Autodesk Inventor part; units mm, degrees
note: some values were not read from the file. Chosen so that the rebuilt part matches the saved one: direction of "Hole2".
(part 16 of 20)
  ellipse E344 centre (-9.843752, -15.647014) end of major axis (-9.7704, -15.822284) minor radius 0.172083 (-9.728588, -15.796415) -> (-9.668946, -15.655192) ccw
  ellipse E345 centre (-10.850532, -15.747299) end of major axis (-10.841654, -15.557507) minor radius 0.073999 (-10.924833, -15.778395) -> (-10.914737, -15.859463) ccw
  ellipse E346 centre (-10.901535, -13.717011) end of major axis (-10.892656, -13.527218) minor radius 0.073999 (-10.972145, -13.675357) -> (-10.975835, -13.748106) ccw
  line L433 (-10.732194, -13.203469) -> (-10.766856, -11.823661)
  line L434 (-10.84586, -11.667497) -> (-11.030789, -11.744892)
  line L435 (-11.144186, -17.767984) -> (-10.697309, -17.58096)
  line L436 (-10.627713, -17.362604) -> (-10.662375, -15.982796)
  line L437 (-10.594189, -13.209925) -> (-10.628851, -11.830117)
  line L438 (-10.489708, -17.369061) -> (-10.52437, -15.989253)
  line L439 (-11.411804, -17.944199) -> (-10.559304, -17.587416)
  ellipse E347 centre (-10.841156, -11.854757) end of major axis (-10.832277, -11.664964) minor radius 0.073999 (-10.766856, -11.823661) -> (-10.84586, -11.667497) ccw
  ellipse E348 centre (-10.702013, -17.3937) end of major axis (-10.710892, -17.583493) minor radius 0.073999 (-10.697309, -17.58096) -> (-10.627713, -17.362604) ccw
  ellipse E349 centre (-10.703151, -11.861213) end of major axis (-10.694272, -11.671421) minor radius 0.073999 (-10.628851, -11.830117) -> (-10.694272, -11.671421) ccw
  ellipse E350 centre (-10.564008, -17.400156) end of major axis (-10.572887, -17.589949) minor radius 0.073999 (-10.559304, -17.587416) -> (-10.489708, -17.369061) ccw
  line L440 (-10.832277, -11.664964) -> (-10.694272, -11.671421)
  line L441 (-10.643313, -18.02564) -> (-11.279559, -17.995875)
  line L442 (-11.338217, -18.020424) -> (-10.641932, -18.052998)
  ellipse E351 centre (-11.181795, -17.954959) end of major axis (-11.431717, -17.961237) minor radius 0.041852 (-11.411804, -17.944199) -> (-11.279559, -17.995875) ccw
  ellipse E352 centre (-11.181795, -17.954959) end of major axis (-11.581669, -17.965004) minor radius 0.066962 (-11.579808, -17.958216) -> (-11.338217, -18.020424) ccw
  line L443 (-11.581818, -17.959094) -> (-11.581669, -17.965004)
  line L444 (9.445486, -13.382673) -> (9.726407, -13.372264)
  line L445 (9.577459, -15.622189) -> (9.444613, -14.35264)
  ellipse E353 centre (9.612924, -11.790422) end of major axis (9.588034, -11.602059) minor radius 0.101721 (9.69231, -11.695037) -> (9.593168, -11.601626) ccw
  line L446 (9.593168, -11.601626) -> (9.489906, -11.605452)
  line L447 (9.680903, -17.583459) -> (9.975636, -17.572538)
  line L448 (9.986075, -17.572152) -> (10.054617, -17.569612)
  line L449 (9.494074, -17.602324) -> (9.600374, -17.598385)
  ellipse E354 centre (9.679434, -15.618411) end of major axis (9.704324, -15.806773) minor radius 0.101721 (9.577459, -15.622189) -> (9.667019, -15.799296) ccw
  ellipse E355 centre (9.465242, -13.571468) end of major axis (9.440352, -13.383106) minor radius 0.101721 (9.445486, -13.382673) -> (9.445133, -13.382687) ccw
  line L450 (-9.369641, -11.620465) -> (-9.45962, -11.620315)
  line L451 (-9.704796, -17.582819) -> (-9.665179, -17.582885)
  line L452 (-9.476199, -17.583199) -> (-9.245372, -17.583582)
  line L453 (-9.152463, -17.394911) -> (-9.079808, -16.701606)
  line L454 (-9.581549, -17.599678) -> (-9.512402, -17.599793)
  ellipse E356 centre (-9.225588, -17.39479) end of major axis (-9.248733, -17.583375) minor radius 0.072673 (-9.245372, -17.583582) -> (-9.152463, -17.394911) ccw
  line L455 (-9.214159, -15.814637) -> (-9.257838, -15.814565)
  ellipse E357 centre (-9.092788, -11.665336) end of major axis (-9.49061, -11.623647) minor radius 0.017093 (-9.45962, -11.620315) -> (-9.49061, -11.623647) ccw
  line L456 (-9.49061, -11.623647) -> (-9.491123, -11.628548)
  line L457 (11.417851, -17.944787) -> (11.028639, -17.977434)
  line L458 (10.650943, -18.039039) -> (11.499343, -17.967874)
  ellipse E358 centre (11.422583, -17.757528) end of major axis (11.370793, -17.940333) minor radius 0.156811 (11.417851, -17.944787) -> (11.502296, -17.909857) ccw
  ellipse E359 centre (11.504076, -17.780615) end of major axis (11.452286, -17.963421) minor radius 0.156811 (11.499343, -17.967874) -> (11.586117, -17.931064) ccw
  line L459 (10.678705, -11.674527) -> (10.647369, -11.665649)
  line L460 (10.497918, -17.579089) -> (10.937664, -17.703672)
  line L461 (10.490349, -17.623165) -> (11.556403, -17.925185)
  line L462 (10.603032, -13.41997) -> (10.918137, -13.509241)
  line L463 (11.016629, -13.725744) -> (10.965317, -15.756025)
  ellipse E360 centre (10.26736, -13.448126) end of major axis (10.667233, -13.458232) minor radius 0.066962 (10.603032, -13.41997) -> (10.37813, -13.386485) ccw
  line L464 (9.644854, -13.420548) -> (9.985302, -13.391991)
  ellipse E361 centre (10.26736, -13.448126) end of major axis (10.01744, -13.44181) minor radius 0.041852 (10.251549, -13.405957) -> (10.137481, -13.409169) ccw
  line L465 (10.633643, -13.474862) -> (10.568229, -13.45633)
  ellipse E362 centre (10.206584, -15.852925) end of major axis (9.806712, -15.842819) minor radius 0.066962 (10.532407, -15.822097) -> (10.256875, -15.787709) ccw
  line L466 (9.547773, -13.645477) -> (9.541369, -13.898884)
  ellipse E363 centre (10.913405, -13.6965) end of major axis (10.897523, -13.507165) minor radius 0.102463 (11.016629, -13.725744) -> (10.918137, -13.509241) ccw
  ellipse E364 centre (10.862093, -15.726781) end of major axis (10.846211, -15.537446) minor radius 0.102463 (10.937384, -15.870856) -> (10.965317, -15.756025) ccw
  ellipse E365 centre (9.707217, -13.632102) end of major axis (9.759007, -13.449297) minor radius 0.156811 (9.558959, -13.580771) -> (9.547773, -13.645477) ccw
  ellipse E366 centre (9.625724, -13.609015) end of major axis (9.573934, -13.79182) minor radius 0.156811 (9.59069, -13.430952) -> (9.493397, -13.520415) ccw
  line L467 (9.339233, -17.62641) -> (9.636108, -17.601507)
  line L468 (9.968091, -17.57366) -> (10.026426, -17.568767)
  ellipse E367 centre (10.162247, -17.607246) end of major axis (10.412167, -17.613562) minor radius 0.041852 (10.171389, -17.565634) -> (10.026426, -17.568767) ccw
  ellipse E368 centre (10.311697, -11.693806) end of major axis (9.911825, -11.6837) minor radius 0.066962 (10.647369, -11.665649) -> (10.343834, -11.627829) ccw
  ellipse E369 centre (10.162247, -17.607246) end of major axis (9.762375, -17.59714) minor radius 0.066962 (10.497918, -17.579089) -> (10.333285, -17.550901) ccw
  ellipse E370 centre (11.561135, -17.737926) end of major axis (11.577017, -17.927261) minor radius 0.102463 (11.556403, -17.925185) -> (11.575565, -17.927364) ccw
  line L469 (9.071223, -17.982215) -> (9.026913, -17.969662)
  ellipse E371 centre (-10.756466, -13.251165) end of major axis (-10.832503, -13.077043) minor radius 0.168992 (-10.928737, -13.245323) -> (-10.838461, -13.407289) ccw
  ellipse E372 centre (-10.819297, -13.278602) end of major axis (-10.74326, -13.452724) minor radius 0.168992 (-10.947502, -13.391229) -> (-10.896969, -13.437563) ccw
  ellipse E373 centre (-11.00923, -13.280047) end of major axis (-11.015669, -13.469938) minor radius 0.079929 (-10.999805, -13.46675) -> (-10.929643, -13.245292) ccw
  ellipse E374 centre (-11.145233, -13.275435) end of major axis (-11.151672, -13.465326) minor radius 0.079929 (-11.135808, -13.462138) -> (-11.065647, -13.240681) ccw
  ellipse E375 centre (-11.005348, -16.0465) end of major axis (-10.998909, -15.856609) minor radius 0.079929 (-10.925762, -16.011746) -> (-11.014773, -15.859797) ccw
  ellipse E376 centre (-10.616581, -16.02223) end of major axis (-10.692618, -15.848108) minor radius 0.168992 (-10.754817, -15.898029) -> (-10.788852, -16.016388) ccw
  ellipse E377 centre (-10.869345, -16.051112) end of major axis (-10.862906, -15.861221) minor radius 0.079929 (-10.789758, -16.016357) -> (-10.862906, -15.861221) ccw
  line L470 (-10.862906, -15.861221) -> (-10.998909, -15.856609)
  line L471 (-10.679739, -13.469718) -> (-10.756571, -13.467113)
  line L472 (-10.691215, -13.439761) -> (-10.615929, -13.442313)
  line L473 (-10.019153, -15.69929) -> (-10.037208, -15.341622)
  line L474 (-10.11165, -13.866954) -> (-10.121338, -13.675036)
  line L475 (-11.395511, -13.575548) -> (-11.135808, -13.462138)
  line L476 (-10.999805, -13.46675) -> (-11.259507, -13.580159)
  line L477 (-12.048956, -13.860901) -> (-11.806008, -13.754808)
  line L478 (-11.716997, -13.906757) -> (-11.614811, -15.93101)
  line L479 (-11.684973, -16.152467) -> (-11.92792, -16.25856)
  line L480 (-11.014773, -15.859797) -> (-11.274475, -15.973207)
  line L481 (-11.363486, -15.821258) -> (-11.465672, -13.797005)
  line L482 (-10.540849, -15.838414) -> (-10.571702, -15.837368)
  line L483 (-11.329669, -13.801617) -> (-11.227483, -15.82587)
  ellipse E378 centre (-11.68628, -13.873199) end of major axis (-12.085772, -13.893366) minor radius 0.071491 (-12.048956, -13.860901) -> (-11.85383, -13.946367) ccw
  line L484 (-11.714759, -13.951082) -> (-11.85383, -13.946367)
  line L485 (-11.790999, -13.918929) -> (-11.733349, -13.920884)
  ellipse E379 centre (-11.68628, -13.873199) end of major axis (-11.935962, -13.885803) minor radius 0.044682 (-11.912952, -13.865513) -> (-11.790999, -13.918929) ccw
  line L486 (-11.743379, -13.791462) -> (-11.912952, -13.865513)
  ellipse E380 centre (-11.565245, -16.270858) end of major axis (-11.964736, -16.291025) minor radius 0.071491 (-11.92792, -16.25856) -> (-11.964736, -16.291025) ccw
  line L487 (-10.058507, -13.647599) -> (-10.044208, -13.930851)
  line L488 (-9.974022, -15.321217) -> (-9.956321, -15.671852)
  ellipse E381 centre (-10.888744, -11.902896) end of major axis (-10.964781, -11.728775) minor radius 0.168992 (-10.964781, -11.728775) -> (-11.018932, -11.768677) ccw
  ellipse E382 centre (-10.609966, -17.425373) end of major axis (-10.533929, -17.599495) minor radius 0.168992 (-10.615379, -17.610884) -> (-10.600541, -17.612076) ccw
  ellipse E383 centre (-10.547135, -17.397936) end of major axis (-10.623172, -17.223814) minor radius 0.168992 (-10.552098, -17.583502) -> (-10.53771, -17.584639) ccw
  ellipse E384 centre (-10.547135, -17.397936) end of major axis (-10.623172, -17.223814) minor radius 0.168992 (-10.719405, -17.392094) -> (-10.702191, -17.465134) ccw
  ellipse E385 centre (-10.825913, -11.875459) end of major axis (-10.90195, -11.701337) minor radius 0.168992 (-10.895835, -11.698825) -> (-10.998183, -11.869617) ccw
  line L489 (-10.964781, -11.728775) -> (-10.90195, -11.701337)
  line L490 (-10.600541, -17.612076) -> (-10.583907, -17.61264)
  line L491 (-10.431975, -17.617792) -> (-9.338389, -17.654875)
  line L492 (-10.719405, -17.392094) -> (-10.788852, -16.016388)
  line L493 (-10.266545, -17.593834) -> (-10.349114, -17.591034)
  line L494 (-10.517241, -17.585333) -> (-10.53771, -17.584639)
  line L495 (-10.661005, -11.694667) -> (-10.643146, -11.695273)
  line L496 (-10.928737, -13.245323) -> (-10.998183, -11.869617)
  ellipse E386 centre (-10.191423, -15.693448) end of major axis (-10.115386, -15.86757) minor radius 0.168992 (-10.03213, -15.779735) -> (-10.019153, -15.69929) ccw
  ellipse E387 centre (-10.293609, -13.669195) end of major axis (-10.217572, -13.843316) minor radius 0.168992 (-10.121338, -13.675036) -> (-10.128707, -13.629799) ccw
  ellipse E388 centre (-11.796583, -13.941511) end of major axis (-11.790144, -13.75162) minor radius 0.079929 (-11.716997, -13.906757) -> (-11.806008, -13.754808) ccw
  ellipse E389 centre (-11.694398, -15.965764) end of major axis (-11.700837, -16.155655) minor radius 0.079929 (-11.684973, -16.152467) -> (-11.614811, -15.93101) ccw
  ellipse E390 centre (-11.2839, -15.786504) end of major axis (-11.290339, -15.976395) minor radius 0.079929 (-11.363486, -15.821258) -> (-11.274475, -15.973207) ccw
  ellipse E391 centre (-11.386086, -13.762251) end of major axis (-11.379647, -13.57236) minor radius 0.079929 (-11.395511, -13.575548) -> (-11.465672, -13.797005) ccw
  ellipse E392 centre (-10.230778, -13.641757) end of major axis (-10.306815, -13.467635) minor radius 0.168992 (-10.058507, -13.647599) -> (-10.064377, -13.608062) ccw
  ellipse E393 centre (-10.128592, -15.66601) end of major axis (-10.204629, -15.491889) minor radius 0.168992 (-9.990742, -15.79073) -> (-9.956321, -15.671852) ccw
  ellipse E394 centre (-11.147897, -15.791116) end of major axis (-11.141458, -15.601225) minor radius 0.079929 (-11.227483, -15.82587) -> (-11.201101, -15.941165) ccw
  ellipse E395 centre (-11.250082, -13.766862) end of major axis (-11.243643, -13.576972) minor radius 0.079929 (-11.259507, -13.580159) -> (-11.329669, -13.801617) ccw
  line L497 (-11.065647, -13.240681) -> (-11.135093, -11.864974)
  line L498 (-11.224104, -11.713026) -> (-12.137252, -12.111789)
  line L499 (-11.839624, -18.007672) -> (-10.926477, -17.608909)
  line L500 (-10.856315, -17.387452) -> (-10.925762, -16.011746)
  line L501 (-10.929643, -13.245292) -> (-10.99909, -11.869586)
  line L502 (-10.720312, -17.392063) -> (-10.789758, -16.016357)
  line L503 (-11.703621, -18.012284) -> (-10.790473, -17.613521)
  ellipse E396 centre (-11.214679, -11.899729) end of major axis (-11.20824, -11.709838) minor radius 0.079929 (-11.135093, -11.864974) -> (-11.224104, -11.713026) ccw
  ellipse E397 centre (-10.935901, -17.422206) end of major axis (-10.94234, -17.612097) minor radius 0.079929 (-10.926477, -17.608909) -> (-10.856315, -17.387452) ccw
  ellipse E398 centre (-11.078676, -11.904341) end of major axis (-11.072237, -11.71445) minor radius 0.079929 (-10.99909, -11.869586) -> (-11.072237, -11.71445) ccw
  ellipse E399 centre (-10.799898, -17.426818) end of major axis (-10.806337, -17.616709) minor radius 0.079929 (-10.790473, -17.613521) -> (-10.720312, -17.392063) ccw
  line L504 (-11.20824, -11.709838) -> (-11.072237, -11.71445)
  line L505 (-10.639678, -18.097642) -> (-11.581668, -18.0657)
  line L506 (-11.644499, -18.093138) -> (-10.638183, -18.127261)
  ellipse E400 centre (-11.476949, -18.01997) end of major axis (-11.726631, -18.032574) minor radius 0.044682 (-11.703621, -18.012284) -> (-11.581668, -18.0657) ccw
  ellipse E401 centre (-11.774577, -12.124087) end of major axis (-12.174068, -12.144254) minor radius 0.071491 (-12.137252, -12.111789) -> (-12.174068, -12.144254) ccw
  ellipse E402 centre (-11.476949, -18.01997) end of major axis (-11.87644, -18.040137) minor radius 0.071491 (-11.839624, -18.007672) -> (-11.644499, -18.093138) ccw
  line L507 (-12.174068, -12.144254) -> (-12.085772, -13.893366)
  line L508 (-11.964736, -16.291025) -> (-11.87644, -18.040137)
  ellipse E403 centre (9.621764, -13.167497) end of major axis (9.645394, -13.356022) minor radius 0.095931 (9.643038, -13.356259) -> (9.717505, -13.160222) ccw
  line L509 (9.645394, -13.356022) -> (9.618841, -13.35935)
  line L510 (9.443815, -13.371397) -> (9.643038, -13.356259)
  line L511 (9.799774, -15.789209) -> (9.60382, -15.804099)
  line L512 (9.486806, -15.622612) -> (9.386714, -14.734494)
  line L513 (9.717505, -13.160222) -> (9.560751, -11.769345)
  line L514 (9.443737, -11.587858) -> (9.2374, -11.603537)
  line L515 (9.01704, -17.632231) -> (9.957912, -17.560738)
  line L516 (8.945553, -17.644004) -> (9.57653, -17.596058)
  ellipse E404 centre (9.46501, -11.77662) end of major axis (9.441381, -11.588095) minor radius 0.095931 (9.560751, -11.769345) -> (9.443737, -11.587858) ccw
  ellipse E405 centre (9.582546, -15.615337) end of major axis (9.606176, -15.803862) minor radius 0.095931 (9.486806, -15.622612) -> (9.60382, -15.804099) ccw
  ellipse E406 centre (8.67445, -17.675171) end of major axis (8.276966, -17.719968) minor radius 0.00852 (9.01704, -17.632231) -> (8.94642, -17.638281) ccw
  line L517 (-9.228619, -11.605746) -> (-9.331213, -11.599017)
  line L518 (-9.855856, -17.569528) -> (-9.103656, -17.618867)
  line L519 (-9.00389, -17.435255) -> (-8.988858, -17.302054)
  line L520 (-9.540587, -17.597944) -> (-8.968083, -17.635496)
  line L521 (-9.530783, -13.367387) -> (-9.435311, -13.373649)
  line L522 (-9.370298, -14.783825) -> (-9.465065, -15.623544)
  line L523 (-9.564831, -15.807156) -> (-9.804351, -15.791446)
  ellipse E407 centre (-9.169255, -13.411732) end of major axis (-9.566732, -13.366875) minor radius 0.00852 (-9.530783, -13.367387) -> (-9.557888, -13.366094) ccw
  ellipse E408 centre (-9.442823, -15.83579) end of major axis (-9.8403, -15.790933) minor radius 0.00852 (-9.804351, -15.791446) -> (-9.8403, -15.790933) ccw
  ellipse E409 centre (-9.543528, -15.618398) end of major axis (-9.56666, -15.806984) minor radius 0.078528 (-9.564831, -15.807156) -> (-9.465065, -15.623544) ccw
  ellipse E410 centre (-9.082354, -17.430108) end of major axis (-9.105486, -17.618695) minor radius 0.078528 (-9.103656, -17.618867) -> (-9.00389, -17.435255) ccw
  ellipse E411 centre (-8.946781, -17.446738) end of major axis (-8.969913, -17.635324) minor radius 0.078528 (-8.968083, -17.635496) -> (-8.939824, -17.625771) ccw
  ellipse E412 centre (-8.969685, -11.643361) end of major axis (-9.367162, -11.598504) minor radius 0.00852 (-9.331213, -11.599017) -> (-9.367162, -11.598504) ccw
  line L524 (-9.367162, -11.598504) -> (-9.370271, -11.626052)
  line L525 (-9.8403, -15.790933) -> (-9.841486, -15.80144)
  ellipse E413 centre (11.975018, -13.723987) end of major axis (11.912145, -13.903283) minor radius 0.159857 (11.965565, -13.910689) -> (12.063067, -13.869699) ccw
  ellipse E414 centre (11.898512, -13.697159) end of major axis (11.835639, -13.876455) minor radius 0.159857 (11.889059, -13.88386) -> (11.979456, -13.848629) ccw
  ellipse E415 centre (12.042124, -13.680589) end of major axis (12.053014, -13.870276) minor radius 0.096916 (12.032671, -13.86729) -> (12.053014, -13.870276) ccw
  ellipse E416 centre (12.170931, -13.673194) end of major axis (12.181821, -13.862882) minor radius 0.096916 (12.161477, -13.859896) -> (12.267838, -13.707176) ccw
  ellipse E417 centre (12.030624, -16.444238) end of major axis (12.019734, -16.25455) minor radius 0.096916 (12.127532, -16.47822) -> (12.040078, -16.257536) ccw
  line L526 (12.181821, -13.862882) -> (12.053014, -13.870276)
  line L527 (11.796803, -13.889157) -> (11.889059, -13.88386)
  line L528 (11.965565, -13.910689) -> (11.749956, -13.923067)
  line L529 (11.845253, -13.749005) -> (12.161477, -13.859896)
  line L530 (12.032671, -13.86729) -> (11.775728, -13.777188)
  line L531 (11.049591, -13.469992) -> (11.345414, -13.573728)
  line L532 (11.432868, -13.794412) -> (11.330375, -15.818649)
  line L533 (11.224014, -15.971368) -> (10.928191, -15.867632)
  line L534 (12.040078, -16.257536) -> (11.723853, -16.146646)
  line L535 (11.636399, -15.925962) -> (11.738892, -13.901725)
  ellipse E418 centre (10.706106, -13.489711) end of major axis (11.105595, -13.509938) minor radius 0.071491 (11.049591, -13.469992) -> (10.616703, -13.415564) ccw
  ellipse E419 centre (10.706106, -13.489711) end of major axis (10.456426, -13.477069) minor radius 0.044682 (10.920784, -13.477386) -> (10.707082, -13.445022) ccw
  line L536 (11.216607, -13.581122) -> (10.920784, -13.477386)
  ellipse E420 centre (10.584706, -15.887352) end of major axis (10.185218, -15.867124) minor radius 0.071491 (10.928191, -15.867632) -> (10.492843, -15.813187) ccw
  line L537 (11.201568, -15.826044) -> (11.304061, -13.801806)
  line L538 (9.800222, -15.612006) -> (9.815689, -15.306536)
  line L539 (9.877415, -14.087452) -> (9.899198, -13.657237)
  line L540 (11.679097, -18.0306) -> (10.648374, -18.089773)
  line L541 (10.646789, -18.121084) -> (11.755603, -18.057428)
  ellipse E421 centre (11.68855, -17.843898) end of major axis (11.625676, -18.023194) minor radius 0.159857 (11.679097, -18.0306) -> (11.769494, -17.995369) ccw
  ellipse E422 centre (11.765056, -17.870726) end of major axis (11.702182, -18.050022) minor radius 0.159857 (11.755603, -18.057428) -> (11.853105, -18.016438) ccw
  line L542 (12.267838, -13.707176) -> (12.337494, -12.331481)
  line L543 (12.25004, -12.110797) -> (11.138153, -11.720893)
  line L544 (10.839628, -17.616731) -> (11.951515, -18.006635)
  line L545 (12.057876, -17.853916) -> (12.127532, -16.47822)
  line L546 (10.710822, -17.624126) -> (11.822709, -18.014029)
  ellipse E423 centre (12.240586, -12.297499) end of major axis (12.229697, -12.107811) minor radius 0.096916 (12.337494, -12.331481) -> (12.25004, -12.110797) ccw
  ellipse E424 centre (11.960969, -17.819933) end of major axis (11.971858, -18.009621) minor radius 0.096916 (11.951515, -18.006635) -> (12.057876, -17.853916) ccw
  ellipse E425 centre (11.832162, -17.827328) end of major axis (11.843052, -18.017016) minor radius 0.096916 (11.822709, -18.014029) -> (11.843052, -18.017016) ccw
  line L547 (11.971858, -18.009621) -> (11.843052, -18.017016)
  ellipse E426 centre (11.33596, -13.760429) end of major axis (11.325071, -13.570741) minor radius 0.096916 (11.432868, -13.794412) -> (11.345414, -13.573728) ccw
  ellipse E427 centre (11.233467, -15.784667) end of major axis (11.244357, -15.974354) minor radius 0.096916 (11.224014, -15.971368) -> (11.330375, -15.818649) ccw
  ellipse E428 centre (11.733306, -15.959945) end of major axis (11.744196, -16.149632) minor radius 0.096916 (11.636399, -15.925962) -> (11.723853, -16.146646) ccw
  ellipse E429 centre (11.8358, -13.935707) end of major axis (11.82491, -13.746019) minor radius 0.096916 (11.845253, -13.749005) -> (11.738892, -13.901725) ccw
  ellipse E430 centre (11.207154, -13.767824) end of major axis (11.196264, -13.578136) minor radius 0.096916 (11.304061, -13.801806) -> (11.216607, -13.581122) ccw
  ellipse E431 centre (10.139788, -13.656348) end of major axis (10.202661, -13.477052) minor radius 0.159857 (9.980403, -13.634911) -> (9.978619, -13.645423) ccw
  ellipse E432 centre (10.063282, -13.62952) end of major axis (10.000409, -13.808815) minor radius 0.159857 (9.90416, -13.606757) -> (9.901654, -13.621935) ccw
  ellipse E433 centre (9.960788, -15.653757) end of major axis (9.897915, -15.833053) minor radius 0.159857 (9.802392, -15.719049) -> (9.83254, -15.784764) ccw
  ellipse E434 centre (10.037294, -15.680585) end of major axis (10.100168, -15.50129) minor radius 0.159857 (9.876569, -15.734065) -> (9.890555, -15.780496) ccw
  ellipse E435 centre (11.10466, -15.792061) end of major axis (11.11555, -15.981749) minor radius 0.096916 (11.164732, -15.95058) -> (11.201568, -15.826044) ccw
  line L548 (9.677127, -17.631435) -> (10.306232, -17.595319)
  line L549 (10.204137, -17.56996) -> (10.003578, -17.581474)
  line L550 (9.653068, -17.601596) -> (9.595968, -17.604874)
  ellipse E436 centre (10.496144, -17.63645) end of major axis (10.745824, -17.649092) minor radius 0.044682 (10.710822, -17.624126) -> (10.579336, -17.598346) ccw
  ellipse E437 centre (10.794669, -11.740612) end of major axis (10.39518, -11.720385) minor radius 0.071491 (11.138153, -11.720893) -> (10.651336, -11.666773) ccw
  ellipse E438 centre (10.496144, -17.63645) end of major axis (10.096656, -17.616223) minor radius 0.071491 (10.839628, -17.616731) -> (10.47045, -17.563759) ccw
  ellipse E439 centre (-10.031545, -13.19179) end of major axis (-9.973156, -13.372596) minor radius 0.167961 (-10.201705, -13.17958) -> (-10.030323, -13.379423) ccw
  ellipse E440 centre (-10.098273, -13.213339) end of major axis (-10.039884, -13.394145) minor radius 0.167961 (-10.228099, -13.324234) -> (-10.097051, -13.400972) ccw
  ellipse E441 centre (-10.080134, -15.998197) end of major axis (-10.138523, -15.817391) minor radius 0.167961 (-10.138523, -15.817391) -> (-10.201976, -15.857572) ccw
  ellipse E442 centre (-10.287123, -13.206811) end of major axis (-10.300722, -13.396324) minor radius 0.083645 (-10.285901, -13.394443) -> (-10.2026, -13.179515) ccw
  ellipse E443 centre (-10.42146, -13.197171) end of major axis (-10.435059, -13.386684) minor radius 0.083645 (-10.420238, -13.384803) -> (-10.336937, -13.169875) ccw
  ellipse E444 centre (-10.403321, -15.982028) end of major axis (-10.389722, -15.792516) minor radius 0.083645 (-10.318798, -15.954733) -> (-10.404543, -15.794396) ccw
  ellipse E445 centre (-10.013406, -15.976648) end of major axis (-10.071795, -15.795842) minor radius 0.167961 (-10.014628, -15.789016) -> (-10.183566, -15.964437) ccw
  ellipse E446 centre (-10.268984, -15.991668) end of major axis (-10.255385, -15.802156) minor radius 0.083645 (-10.184461, -15.964373) -> (-10.255385, -15.802156) ccw
  line L551 (-10.071795, -15.795842) -> (-10.138523, -15.817391)
  line L552 (-10.255385, -15.802156) -> (-10.389722, -15.792516)
  line L553 (-9.596422, -13.436897) -> (-10.097051, -13.400972)
  line L554 (-10.030323, -13.379423) -> (-9.529694, -13.415348)
  line L555 (-10.696048, -13.473872) -> (-10.682857, -13.469612)
  line L556 (-10.681518, -13.46918) -> (-10.420238, -13.384803)
  line L557 (-10.285901, -13.394443) -> (-10.456104, -13.449408)
  line L558 (-10.404543, -15.794396) -> (-10.558715, -15.844184)
  line L559 (-10.766099, -15.723128) -> (-10.774361, -14.454574)
  line L560 (-10.777236, -14.013288) -> (-10.779349, -13.6888)
  line L561 (-9.75757, -15.807462) -> (-10.014628, -15.789016)
  line L562 (-10.645012, -13.69844) -> (-10.643342, -13.954818)
  line L563 (-10.634006, -15.388151) -> (-10.631762, -15.732769)
  ellipse E447 centre (-10.107278, -11.830786) end of major axis (-10.165667, -11.64998) minor radius 0.167961 (-10.165667, -11.64998) -> (-10.22912, -11.690161) ccw
  ellipse E448 centre (-10.071129, -17.38075) end of major axis (-10.012741, -17.561556) minor radius 0.167961 (-10.200955, -17.491645) -> (-10.069907, -17.568383) ccw
  ellipse E449 centre (-10.004401, -17.359201) end of major axis (-9.946012, -17.540007) minor radius 0.167961 (-10.174561, -17.346991) -> (-10.003179, -17.546834) ccw
  ellipse E450 centre (-10.04055, -11.809237) end of major axis (-10.098938, -11.628431) minor radius 0.167961 (-10.041772, -11.621605) -> (-10.21071, -11.797026) ccw
  line L564 (-10.165667, -11.64998) -> (-10.098938, -11.628431)
  line L565 (-10.069907, -17.568383) -> (-9.882923, -17.581801)
  line L566 (-9.62212, -17.600516) -> (-9.24945, -17.627259)
  line L567 (-10.174561, -17.346991) -> (-10.183566, -15.964437)
  line L568 (-9.826429, -17.559517) -> (-10.003179, -17.546834)
  line L569 (-10.041772, -11.621605) -> (-9.593855, -11.653747)
  line L570 (-10.201705, -13.17958) -> (-10.21071, -11.797026)
  ellipse E451 centre (-9.5952, -13.624529) end of major axis (-9.653589, -13.443723) minor radius 0.167961 (-9.453768, -13.531516) -> (-9.596422, -13.436897) ccw
  ellipse E452 centre (-10.681576, -15.695833) end of major axis (-10.695175, -15.885346) minor radius 0.083645 (-10.766099, -15.723128) -> (-10.754244, -15.813011) ccw
  ellipse E453 centre (-10.694826, -13.661504) end of major axis (-10.681227, -13.471992) minor radius 0.083645 (-10.696048, -13.473872) -> (-10.710578, -13.48137) ccw
  ellipse E454 centre (-10.694826, -13.661504) end of major axis (-10.708426, -13.851017) minor radius 0.083645 (-10.772841, -13.611804) -> (-10.779349, -13.6888) ccw
  ellipse E455 centre (-9.528472, -13.60298) end of major axis (-9.58686, -13.422174) minor radius 0.167961 (-9.474177, -13.429569) -> (-9.529694, -13.415348) ccw
  ellipse E456 centre (-10.547239, -15.705473) end of major axis (-10.53364, -15.51596) minor radius 0.083645 (-10.631762, -15.732769) -> (-10.626023, -15.796522) ccw
  ellipse E457 centre (-10.560489, -13.671145) end of major axis (-10.54689, -13.481632) minor radius 0.083645 (-10.638486, -13.62134) -> (-10.645012, -13.69844) ccw
  line L571 (-10.336937, -13.169875) -> (-10.345942, -11.787322)
  line L572 (-10.431687, -11.626985) -> (-10.657434, -11.699887)
  line L573 (-10.752585, -17.668307) -> (-10.393094, -17.552214)
  line L574 (-10.309793, -17.337287) -> (-10.318798, -15.954733)
  line L575 (-10.2026, -13.179515) -> (-10.211605, -11.796962)
  line L576 (-10.175456, -17.346927) -> (-10.184461, -15.964373)
  line L577 (-11.228543, -17.875033) -> (-10.258757, -17.561854)
  ellipse E458 centre (-10.430465, -11.814617) end of major axis (-10.416865, -11.625105) minor radius 0.083645 (-10.345942, -11.787322) -> (-10.431687, -11.626985) ccw
  ellipse E459 centre (-10.394316, -17.364582) end of major axis (-10.407915, -17.554095) minor radius 0.083645 (-10.393094, -17.552214) -> (-10.309793, -17.337287) ccw
  ellipse E460 centre (-10.296128, -11.824257) end of major axis (-10.282529, -11.634745) minor radius 0.083645 (-10.211605, -11.796962) -> (-10.282529, -11.634745) ccw
  ellipse E461 centre (-10.259979, -17.374222) end of major axis (-10.273578, -17.563735) minor radius 0.083645 (-10.258757, -17.561854) -> (-10.175456, -17.346927) ccw
  line L578 (-10.416865, -11.625105) -> (-10.282529, -11.634745)
  line L579 (-10.993106, -17.935823) -> (-11.115863, -17.927014)
  line L580 (-11.182591, -17.948563) -> (-10.961458, -17.964432)
  ellipse E462 centre (-11.004649, -17.891099) end of major axis (-11.254643, -17.892728) minor radius 0.039312 (-11.228543, -17.875033) -> (-11.115863, -17.927014) ccw
  ellipse E463 centre (-11.004649, -17.891099) end of major axis (-10.604657, -17.888494) minor radius 0.062899 (-11.359601, -17.922351) -> (-11.182591, -17.948563) ccw
  line L581 (9.569097, -13.392619) -> (9.66923, -13.393144)
  line L582 (9.560898, -13.410165) -> (9.53155, -13.410011)
  line L583 (9.69419, -15.627786) -> (9.494388, -13.58092)
  ellipse E464 centre (9.718804, -11.81435) end of major axis (9.694287, -11.625939) minor radius 0.092496 (9.718615, -11.629173) -> (9.700376, -11.625561) ccw
  ellipse E465 centre (10.133966, -17.415425) end of major axis (10.158483, -17.603837) minor radius 0.092496 (10.152394, -17.604214) -> (10.158483, -17.603837) ccw
  line L584 (10.15897, -17.603773) -> (10.158483, -17.603837)
  line L585 (9.700376, -11.625561) -> (9.647072, -11.625282)
  line L586 (9.712882, -17.584322) -> (10.015932, -17.58591)
  line L587 (9.530976, -17.600956) -> (9.91367, -17.602962)
  line L588 (10.151389, -17.604208) -> (10.152394, -17.604214)
  ellipse E466 centre (9.787328, -15.628274) end of major axis (9.811845, -15.816685) minor radius 0.092496 (9.69419, -15.627786) -> (9.756335, -15.791118) ccw
  ellipse E467 centre (9.587526, -13.581408) end of major axis (9.563009, -13.392996) minor radius 0.092496 (9.569097, -13.392619) -> (9.494388, -13.58092) ccw
  line L589 (-9.364516, -11.625933) -> (-9.601494, -11.630827)
  line L590 (-9.934587, -17.587325) -> (-9.692602, -17.582328)
  line L591 (-9.826588, -17.604738) -> (-9.571711, -17.599475)
  line L592 (-9.659339, -13.397075) -> (-9.51984, -13.394194)
  line L593 (-9.493169, -13.972646) -> (-9.655017, -15.628093)
  line L594 (-9.484689, -13.413112) -> (-9.525115, -13.413947)
  ellipse E468 centre (-9.538297, -13.58298) end of major axis (-9.514553, -13.39447) minor radius 0.082693 (-9.453149, -13.526216) -> (-9.51984, -13.394194) ccw
  ellipse E469 centre (-9.73841, -15.629816) end of major axis (-9.714667, -15.441305) minor radius 0.082693 (-9.716936, -15.797179) -> (-9.655017, -15.628093) ccw
  ellipse E470 centre (-9.244188, -11.67583) end of major axis (-9.64229, -11.636909) minor radius 0.022991 (-9.601494, -11.630827) -> (-9.64229, -11.636909) ccw
  line L595 (-9.64229, -11.636909) -> (-9.643588, -11.650178)
  line L596 (11.185193, -17.903366) -> (11.02199, -17.916975)
  line L597 (11.026254, -17.943789) -> (11.25963, -17.924328)
  ellipse E471 centre (11.186443, -17.715734) end of major axis (11.134941, -17.89862) minor radius 0.162803 (11.185193, -17.903366) -> (11.272843, -17.867526) ccw
  ellipse E472 centre (11.26088, -17.736696) end of major axis (11.209378, -17.919583) minor radius 0.162803 (11.25963, -17.924328) -> (11.319457, -17.906607) ccw
  line L598 (10.407344, -13.401032) -> (10.586269, -13.451419)
  line L599 (10.788203, -13.69627) -> (10.774643, -15.730597)
  ellipse E473 centre (10.060081, -13.42999) end of major axis (10.460072, -13.432656) minor radius 0.062899 (10.407344, -13.401032) -> (9.861582, -13.374091) ccw
  line L600 (9.660929, -13.390823) -> (9.861582, -13.374091)
  line L601 (9.936019, -13.395053) -> (9.516949, -13.429998)
  ellipse E474 centre (10.060081, -13.42999) end of major axis (9.810087, -13.428324) minor radius 0.039312 (10.27712, -13.411891) -> (9.936019, -13.395053) ccw
  line L602 (10.438719, -13.457399) -> (10.27712, -13.411891)
  line L603 (9.845521, -15.783681) -> (9.730643, -15.793261)
  ellipse E475 centre (10.04402, -15.839581) end of major axis (9.644029, -15.836914) minor radius 0.062899 (10.350877, -15.801227) -> (9.845521, -15.783681) ccw
  line L604 (10.64442, -15.741456) -> (10.647429, -15.29004)
  line L605 (10.654815, -14.181942) -> (10.65798, -13.707129)
  ellipse E476 centre (10.693916, -13.669718) end of major axis (10.678127, -13.480375) minor radius 0.093287 (10.788203, -13.69627) -> (10.780265, -13.616226) ccw
  ellipse E477 centre (10.680356, -15.704045) end of major axis (10.664567, -15.514702) minor radius 0.093287 (10.757698, -15.831309) -> (10.774643, -15.730597) ccw
  ellipse E478 centre (10.563693, -13.680577) end of major axis (10.579482, -13.86992) minor radius 0.093287 (10.65798, -13.707129) -> (10.653748, -13.647826) ccw
  ellipse E479 centre (10.550133, -15.714904) end of major axis (10.565922, -15.904247) minor radius 0.093287 (10.644148, -15.753371) -> (10.64442, -15.741456) ccw
  ellipse E480 centre (10.550133, -15.714904) end of major axis (10.565922, -15.904247) minor radius 0.093287 (10.634919, -15.8188) -> (10.642621, -15.775126) ccw
  line L606 (10.379566, -17.568439) -> (10.532831, -17.6116)
  line L607 (10.249342, -17.579298) -> (11.331161, -17.883949)
  line L608 (9.873299, -11.616274) -> (9.655944, -11.634399)
  ellipse E481 centre (10.032303, -17.597397) end of major axis (10.282298, -17.599063) minor radius 0.039312 (10.249342, -17.579298) -> (9.915356, -17.56189) ccw
  ellipse E482 centre (10.071798, -11.672174) end of major axis (9.671807, -11.669508) minor radius 0.062899 (10.398842, -11.638085) -> (9.873299, -11.616274) ccw
  ellipse E483 centre (10.032303, -17.597397) end of major axis (9.632312, -17.594731) minor radius 0.062899 (10.379566, -17.568439) -> (9.837919, -17.541159) ccw
  ellipse E484 centre (11.332411, -17.696317) end of major axis (11.3482, -17.88566) minor radius 0.093287 (11.331161, -17.883949) -> (11.3482, -17.88566) ccw
  line L609 (11.401267, -17.881234) -> (11.3482, -17.88566)
  ellipse E485 centre (-10.024286, -17.752092) end of major axis (-10.466646, -17.763205) minor radius 0.074077 (-10.187129, -17.687172) -> (-10.250815, -17.693976) ccw
  ellipse E486 centre (-10.174025, -17.713677) end of major axis (-10.024073, -17.70991) minor radius 0.025111 (-10.250815, -17.693976) -> (-10.31203, -17.70722) ccw
  ellipse E487 centre (-10.558431, -17.874556) end of major axis (-10.708383, -17.878323) minor radius 0.025111 (-10.696436, -17.8681) -> (-10.7083, -17.87737) ccw
  ellipse E488 centre (-10.524839, -17.887682) end of major axis (-10.674792, -17.891449) minor radius 0.025111 (-10.6523, -17.904026) -> (-10.649418, -17.904705) ccw
  line L610 (-10.696436, -17.8681) -> (-10.646494, -17.847198)
  line L611 (-10.542988, -17.803879) -> (-10.509871, -17.790019)
  line L612 (-10.338718, -17.71839) -> (-10.31203, -17.70722)
  line L613 (-9.074103, -17.792735) -> (-9.133298, -17.817509)
  ellipse E489 centre (-9.855609, -17.818004) end of major axis (-9.275792, -17.803439) minor radius 0.097095 (-9.874411, -17.721389) -> (-10.317705, -17.77062) ccw
  ellipse E490 centre (-10.349627, -17.734493) end of major axis (-10.199818, -17.72693) minor radius 0.026809 (-10.367725, -17.708731) -> (-10.37917, -17.709621) ccw
  ellipse E491 centre (-10.349627, -17.734493) end of major axis (-10.199818, -17.72693) minor radius 0.026809 (-10.313837, -17.706679) -> (-10.323775, -17.70679) ccw
  ellipse E492 centre (-10.433803, -17.744156) end of major axis (-10.283993, -17.736594) minor radius 0.026809 (-10.506513, -17.72424) -> (-10.569806, -17.739544) ccw
  ellipse E493 centre (-10.845555, -17.923965) end of major axis (-10.995364, -17.931527) minor radius 0.026809 (-10.981558, -17.919353) -> (-10.992429, -17.936435) ccw
  ellipse E494 centre (-10.814578, -17.937533) end of major axis (-10.964387, -17.945095) minor radius 0.026809 (-10.945566, -17.956961) -> (-10.877409, -17.96497) ccw
  line L614 (-10.996068, -17.91758) -> (-10.995364, -17.931527)
  ellipse E495 centre (-10.292017, -17.782992) end of major axis (-10.733954, -17.805302) minor radius 0.079087 (-10.37917, -17.709621) -> (-10.506513, -17.72424) ccw
  ellipse E496 centre (-10.559152, -17.899648) end of major axis (-11.001089, -17.921957) minor radius 0.079087 (-10.992429, -17.936435) -> (-10.945566, -17.956961) ccw
  line L615 (-10.981558, -17.919353) -> (-10.569806, -17.739544)
  line L616 (-10.64598, -17.972818) -> (-10.877409, -17.96497)
  ellipse E497 centre (-10.136467, -17.851124) end of major axis (-10.715729, -17.880365) minor radius 0.103663 (-10.110281, -17.74616) -> (-10.648408, -17.92471) ccw
  ellipse E498 centre (10.849847, -17.927701) end of major axis (10.700039, -17.920116) minor radius 0.026809 (10.926353, -17.954529) -> (10.987627, -17.944994) ccw
  ellipse E499 centre (10.871988, -17.913213) end of major axis (11.021796, -17.920798) minor radius 0.026809 (11.021122, -17.923076) -> (11.000795, -17.905818) ccw
  ellipse E500 centre (10.370621, -17.737399) end of major axis (10.520429, -17.744984) minor radius 0.026809 (10.499427, -17.730004) -> (10.429451, -17.715596) ccw
  ellipse E501 centre (10.283702, -17.729172) end of major axis (10.433511, -17.736757) minor radius 0.026809 (10.215629, -17.701924) -> (10.207197, -17.702344) ccw
  line L617 (11.021796, -17.920798) -> (11.022687, -17.903209)
  ellipse E502 centre (10.581176, -17.893978) end of major axis (11.02311, -17.916355) minor radius 0.079087 (10.987627, -17.944994) -> (11.021122, -17.923076) ccw
  ellipse E503 centre (10.255901, -17.779915) end of major axis (9.813967, -17.757538) minor radius 0.079087 (10.429451, -17.715596) -> (10.377649, -17.70976) ccw
  line L618 (10.499427, -17.730004) -> (11.000795, -17.905818)
  line L619 (9.924361, -17.718581) -> (9.927437, -17.718404)
  line L620 (10.142861, -17.706037) -> (10.207197, -17.702344)
  line L621 (10.926353, -17.954529) -> (10.654432, -17.97014)
  ellipse E504 centre (10.14472, -17.852666) end of major axis (10.723978, -17.881996) minor radius 0.103663 (10.65665, -17.92633) -> (10.11855, -17.747698) ccw
  line L622 (9.01994, -17.898228) -> (9.140757, -17.938822)
  ellipse E505 centre (8.531424, -18.083924) end of major axis (9.108736, -18.028144) minor radius 0.148512 (9.107704, -18.041572) -> (9.0262, -17.96236) ccw
  line L623 (-9.13252, -17.93696) -> (-9.010565, -17.885304)
  ellipse E506 centre (-8.523207, -18.082627) end of major axis (-9.10051, -18.026759) minor radius 0.148512 (-9.017964, -17.960988) -> (-9.099479, -18.040188) ccw
  ellipse E507 centre (-9.84173, -17.684518) end of major axis (-9.691733, -17.683541) minor radius 0.023587 (-9.775002, -17.662969) -> (-9.867144, -17.661433) ccw
  ellipse E508 centre (-9.926851, -17.68956) end of major axis (-9.776854, -17.688583) minor radius 0.023587 (-9.995916, -17.66906) -> (-10.061187, -17.67992) ccw
  ellipse E509 centre (-9.792173, -17.729535) end of major axis (-10.234664, -17.732417) minor radius 0.069582 (-9.867144, -17.661433) -> (-9.995916, -17.66906) ccw
  line L624 (-10.130994, -17.702463) -> (-10.061187, -17.67992)
  line L625 (-9.005895, -17.837537) -> (-9.132901, -17.878551)
  line L626 (-9.775002, -17.662969) -> (-8.994305, -17.718992)
  ellipse E510 centre (-9.64845, -17.795837) end of major axis (-9.068463, -17.792059) minor radius 0.091204 (-9.133188, -17.834433) -> (-10.134923, -17.749266) ccw
  ellipse E511 centre (9.183719, -17.674525) end of major axis (9.034428, -17.689098) minor radius 0.008622 (9.31459, -17.665962) -> (9.319759, -17.664858) ccw
  ellipse E512 centre (9.183719, -17.674525) end of major axis (9.034428, -17.689098) minor radius 0.008622 (9.257248, -17.674911) -> (9.259521, -17.674613) ccw
  ellipse E513 centre (9.207596, -17.667205) end of major axis (9.356886, -17.652632) minor radius 0.008622 (9.35588, -17.653783) -> (9.337525, -17.650297) ccw
  line L627 (9.356886, -17.652632) -> (9.354204, -17.625154)
  ellipse E514 centre (8.918441, -17.693376) end of major axis (9.358848, -17.650386) minor radius 0.025434 (9.319759, -17.664858) -> (9.35588, -17.653783) ccw
  line L628 (8.94491, -17.64824) -> (9.337525, -17.650297)
  line L629 (9.257248, -17.674911) -> (9.001391, -17.708204)
  ellipse E515 centre (8.485924, -17.728498) end of major axis (9.063181, -17.67215) minor radius 0.033337 (8.999978, -17.693726) -> (8.942584, -17.663581) ccw
  line L630 (-9.323127, -17.652344) -> (-8.937006, -17.64437)
  line L631 (-8.993195, -17.707638) -> (-9.226122, -17.6783)
  ellipse E516 centre (-9.189138, -17.66922) end of major axis (-9.338426, -17.654625) minor radius 0.008622 (-9.323127, -17.652344) -> (-9.336159, -17.656399) ccw
  ellipse E517 centre (-9.160285, -17.676941) end of major axis (-9.309574, -17.662345) minor radius 0.008622 (-9.292511, -17.668078) -> (-9.226122, -17.6783) ccw
  line L632 (-9.336735, -17.637332) -> (-9.338426, -17.654625)
  ellipse E518 centre (-8.902446, -17.694222) end of major axis (-9.342846, -17.651165) minor radius 0.025434 (-9.336159, -17.656399) -> (-9.292511, -17.668078) ccw
  ellipse E519 centre (-8.477653, -17.727208) end of major axis (-9.0549, -17.670772) minor radius 0.033337 (-8.934302, -17.662221) -> (-8.991701, -17.692358) ccw
  line L633 (10.024858, -17.677581) -> (10.201877, -17.727432)
  line L634 (10.329395, -17.763342) -> (10.337922, -17.765743)
  line L635 (9.002945, -17.724125) -> (9.733555, -17.663201)
  line L636 (9.141179, -17.875523) -> (9.014234, -17.839774)
  ellipse E520 centre (9.894634, -17.68844) end of major axis (10.044631, -17.68944) minor radius 0.023587 (10.024858, -17.677581) -> (9.95583, -17.667303) ccw
  ellipse E521 centre (9.807992, -17.684163) end of major axis (9.957989, -17.685163) minor radius 0.023587 (9.824755, -17.660832) -> (9.733555, -17.663201) ccw
  ellipse E522 centre (9.775303, -17.729659) end of major axis (9.332813, -17.726709) minor radius 0.069582 (9.95583, -17.667303) -> (9.824755, -17.660832) ccw
  ellipse E523 centre (9.656712, -17.797305) end of major axis (9.076725, -17.793439) minor radius 0.091204 (10.143192, -17.750808) -> (9.141443, -17.835823) ccw
  line L637 (-10.577673, -15.786424) -> (-10.603615, -15.797282)
  line L638 (-10.644936, -13.710156) -> (-10.629987, -13.7039)
  line L639 (-10.531671, -15.788576) -> (-10.556305, -15.798886)
  line L640 (-10.577673, -15.786424) -> (-10.580186, -15.686388)
  ellipse E524 centre (-10.482422, -15.645473) end of major axis (-10.470739, -15.395746) minor radius 0.097367 (-10.488612, -15.399079) -> (-10.580186, -15.686388) ccw
  line L641 (-10.488612, -15.399079) -> (-10.13877, -15.252665)
  line L642 (-10.10214, -15.137741) -> (-10.132098, -13.945193)
  line L643 (-10.173679, -13.863001) -> (-10.395069, -13.955656)
  ellipse E525 centre (-10.529711, -13.763021) end of major axis (-10.518028, -13.513294) minor radius 0.097367 (-10.627474, -13.803936) -> (-10.606018, -13.938519) ccw
  line L644 (-10.627474, -13.803936) -> (-10.629987, -13.7039)
  line L645 (-10.086096, -13.947345) -> (-10.056138, -15.139893)
  line L646 (-10.583986, -13.706052) -> (-10.581473, -13.806088)
  ellipse E526 centre (-10.483709, -13.765173) end of major axis (-10.495392, -14.0149) minor radius 0.097367 (-10.581473, -13.806088) -> (-10.566039, -13.92106) ccw
  line L647 (-10.092768, -15.254817) -> (-10.44261, -15.401231)
  ellipse E527 centre (-10.43642, -15.647625) end of major axis (-10.424738, -15.397898) minor radius 0.097367 (-10.44261, -15.401231) -> (-10.534184, -15.68854) ccw
  line L648 (-10.534184, -15.68854) -> (-10.531671, -15.788576)
  line L649 (-10.629987, -13.7039) -> (-10.583986, -13.706052)
  line L650 (-10.531671, -15.788576) -> (-10.577673, -15.786424)
  ellipse E528 centre (-10.141245, -15.154107) end of major axis (-10.145919, -15.253998) minor radius 0.038947 (-10.13877, -15.252665) -> (-10.10214, -15.137741) ccw
  ellipse E529 centre (-10.171203, -13.961559) end of major axis (-10.16653, -13.861668) minor radius 0.038947 (-10.132098, -13.945193) -> (-10.173679, -13.863001) ccw
  ellipse E530 centre (-10.095244, -15.156259) end of major axis (-10.099917, -15.25615) minor radius 0.038947 (-10.092768, -15.254817) -> (-10.056138, -15.139893) ccw
  ellipse E531 centre (-10.125201, -13.963711) end of major axis (-10.120528, -13.86382) minor radius 0.038947 (-10.086096, -13.947345) -> (-10.120528, -13.86382) ccw
  line L651 (-10.16653, -13.861668) -> (-10.120528, -13.86382)
  line L652 (9.921404, -15.728316) -> (9.871517, -15.7325)
  line L653 (9.974036, -13.645799) -> (9.946999, -13.648067)
  line L654 (9.878034, -15.741928) -> (9.948568, -15.736011)
  ellipse E532 centre (10.132046, -15.461825) end of major axis (10.200191, -15.221292) minor radius 0.20633 (9.929117, -15.423146) -> (9.926295, -15.534785) ccw
  ellipse E533 centre (10.172074, -13.878009) end of major axis (10.240219, -13.637475) minor radius 0.20633 (9.969145, -13.839329) -> (9.966323, -13.950969) ccw
  spline S14 degree 3 poles (10.354436, -15.454672) (10.3538, -15.44885) (10.352536, -15.437267) (10.349307, -15.420171) (10.345159, -15.403471) (10.340036, -15.387235) (10.333999, -15.371521) (10.327081, -15.356388) (10.319322, -15.341896) (10.310759, -15.328104) (10.301431, -15.315073) (10.291374, -15.302862) (10.280627, -15.29153) (10.269226, -15.281139) (10.257213, -15.271742) (10.244611, -15.263429) (10.231504, -15.256149) (10.22233, -15.2523) (10.217756, -15.25038) knots 0 0 0 0 0.0680148 0.13532856 0.20193874 0.26783312 0.33299287 0.39739576 0.46101961 0.52384586 0.58586341 0.64707277 0.70749045 0.76715357 0.82612483 0.88449738 0.9423997 1 1 1 1
  spline S15 degree 3 poles (10.083988, -15.257275) (10.079998, -15.2593) (10.072005, -15.263356) (10.060553, -15.270471) (10.049508, -15.278292) (10.038931, -15.286855) (10.028834, -15.296096) (10.019244, -15.305979) (10.010181, -15.316461) (10.001669, -15.327499) (9.99373, -15.339052) (9.986388, -15.351078) (9.979665, -15.363535) (9.973586, -15.376382) (9.968169, -15.389575) (9.963455, -15.403076) (9.959397, -15.416831) (9.95732, -15.426168) (9.956281, -15.430841) knots 0 0 0 0 0.06018783 0.12057167 0.18123059 0.24222053 0.30357693 0.36531731 0.42744398 0.48994661 0.55280476 0.61599027 0.67946962 0.74320611 0.8071621 0.87130105 0.93558968 1 1 1 1
  spline S16 degree 3 poles (9.929117, -15.423146) (9.930312, -15.418538) (9.932703, -15.409318) (9.937532, -15.39584) (9.943211, -15.382664) (9.949786, -15.369842) (9.957185, -15.357396) (9.965372, -15.345359) (9.974297, -15.333758) (9.983916, -15.322624) (9.994183, -15.311985) (10.005053, -15.301872) (10.016481, -15.292313) (10.028422, -15.28334) (10.040829, -15.274976) (10.053664, -15.26727) (10.066853, -15.260186) (10.075932, -15.256057) (10.080468, -15.253994) knots 0 0 0 0 0.06075211 0.12157744 0.18258462 0.24385247 0.30543277 0.36735321 0.42962038 0.49222284 0.55513405 0.61831518 0.68171776 0.7452863 0.80896074 0.87267882 0.93637843 1 1 1 1
  spline S17 degree 3 poles (10.185772, -15.231872) (10.192996, -15.232187) (10.207444, -15.232816) (10.228869, -15.23655) (10.249628, -15.242385) (10.269328, -15.250358) (10.287657, -15.260216) (10.304559, -15.271802) (10.320041, -15.284968) (10.334108, -15.29957) (10.346769, -15.315463) (10.35803, -15.332508) (10.3679, -15.350563) (10.376385, -15.369489) (10.3835, -15.389147) (10.389218, -15.409403) (10.393669, -15.430104) (10.395485, -15.444127) (10.396395, -15.451152) knots 0 0 0 0 0.06486953 0.12974803 0.19473343 0.25817972 0.32016794 0.38123591 0.44183715 0.50233531 0.56300447 0.62403408 0.68553703 0.7475595 0.8100912 0.87307551 0.93641898 1 1 1 1
  spline S18 degree 3 poles (10.393562, -15.563241) (10.392312, -15.569508) (10.389847, -15.581865) (10.38404, -15.599639) (10.376827, -15.616407) (10.368131, -15.632106) (10.358059, -15.646702) (10.346673, -15.660154) (10.334045, -15.672425) (10.320247, -15.683477) (10.305349, -15.693273) (10.289421, -15.701775) (10.272532, -15.708947) (10.254754, -15.71475) (10.236155, -15.719156) (10.216805, -15.722096) (10.196768, -15.723658) (10.183207, -15.72343) (10.176334, -15.723314) knots 0 0 0 0 0.06465055 0.1274876 0.18889307 0.24923877 0.30888211 0.36816237 0.42739777 0.48688361 0.54689159 0.60767024 0.6694463 0.73242683 0.79680187 0.8627473 0.93042784 1 1 1 1
  spline S19 degree 3 poles (10.071892, -15.7007) (10.067208, -15.698688) (10.057893, -15.694689) (10.04443, -15.687787) (10.031487, -15.680296) (10.019121, -15.672172) (10.007353, -15.663454) (9.996216, -15.654163) (9.985739, -15.644321) (9.975953, -15.633952) (9.966886, -15.623079) (9.95857, -15.611724) (9.951034, -15.59991) (9.94431, -15.587661) (9.938423, -15.575001) (9.933424, -15.561948) (9.929258, -15.548542) (9.927285, -15.539381) (9.926295, -15.534785) knots 0 0 0 0 0.06647427 0.13218355 0.19716033 0.2614393 0.32505872 0.38806176 0.45049795 0.51242459 0.57390817 0.63502578 0.69586647 0.75653236 0.81713976 0.87781985 0.93871923 1 1 1 1
  spline S20 degree 3 poles (9.953459, -15.542481) (9.954071, -15.545937) (9.955288, -15.552819) (9.957791, -15.562961) (9.960757, -15.572891) (9.964216, -15.582595) (9.968137, -15.592067) (9.973952, -15.604357) (9.982299, -15.619121) (9.993884, -15.635801) (10.006902, -15.651336) (10.021113, -15.665782) (10.031521, -15.674363) (10.036722, -15.678652) knots 0 0 0 0 0.0644506 0.12832403 0.1917227 0.2547379 0.31744987 0.37992792 0.50437187 0.62845768 0.75238919 0.87624484 1 1 1 1